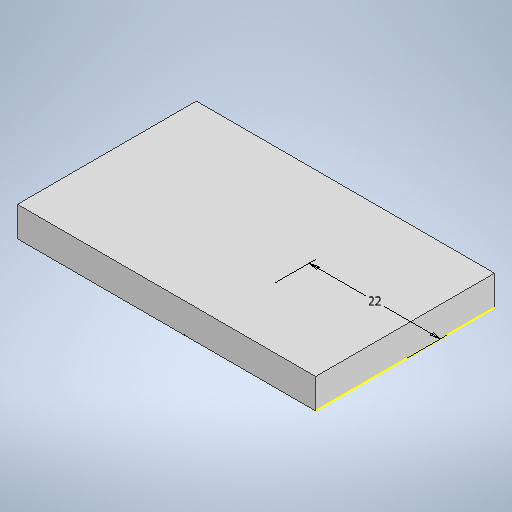
# Autodesk Inventor part: nanoMount
Saved by Autodesk Inventor 2025.1 (Build 291241020, 241B)
## iProperties
Created: 2025-04-14
Part Number: nanoMount
Material: Generic
Document SubType Name: Modeling
Designer: omiye
Density: 1 g/cm^3
Appearance: Default
Author: omiye
Autodesk Inventor part; units mm, degrees
ref_plane "YZ Plane" through (0, 0, 0) normal (1, 0, 0) x (0, 1, 0)
ref_plane "XZ Plane" through (0, 0, 0) normal (0, 1, 0) x (-1, 0, 0)
ref_plane "XY Plane" through (0, 0, 0) normal (0, 0, 1) x (1, 0, 0)
sketch "Sketch1" plane through (0, 0, 0) normal (0, 1, 0) x (-1, 0, 0)
  line L0 (-25, -15) -> (25, -15)
  line L1 (25, -15) -> (25, 15)
  line L2 (25, 15) -> (-25, 15)
  line L3 (-25, 15) -> (-25, -15)
  line L4 (-25, -15) -> (25, 15) construction
  line L5 (25, -15) -> (-25, 15) construction
  point P0 (0, 0)
  dimension "d0" = 50
  dimension "d1" = 30
  constraints: 12 end point, 2 midpoint, 2 parallel, 1 horizontal, 1 perpendicular
  measures "d0" distance of L2.end L1.end
  measures "d1" distance of L1.end L0.end
extrude "Extrusion1" add sketch "Sketch1" along normal blind 5
sketch "Sketch2" plane through (0, 0, 0) normal (0, -1, 0) x (1, 0, 0)
  line L0 (25, 15) -> (25, -15) projected
  line L1 (25, 0) -> (0, 0)
  line L2 (25, 0) -> (3, 0)
  line L3 (3, 0) -> (3, -15)
  line L4 (25, -15) -> (-25, -15) projected
  line L5 (3, 0) -> (3, 15)
  dimension "d4" = 22
  constraints: 8 end point, 3 point on line, 1 horizontal, 1 midpoint, 1 perpendicular
  measures "d4" distance of L1.start L2.end
body "Solid1"
